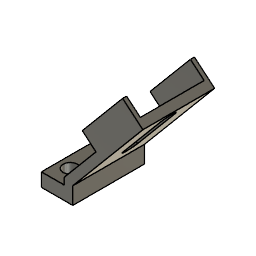
speed_sensor_holder_front_2026 (Autodesk Fusion 360 design; units mm, degrees)
part number: 2026-03-24-16-21-24-312
Autodesk Fusion 360 part; units mm, degrees
sketch "Sketch2" plane through (0, 0, 0) normal (0, 0, 1) x (1, 0, 0)
  line L0 (-7.5122, 7.9259) -> (-0.5122, 7.9259)
  line L1 (-0.5122, 7.9259) -> (-0.5122, -8.0741)
  line L2 (-0.5122, -8.0741) -> (-7.5122, -8.0741)
  line L3 (-7.5122, -8.0741) -> (-7.5122, 7.9259)
  dimension "d1" = 7
  dimension "d2" = 16
  constraint horizontal L0
  constraint vertical L1
  constraint horizontal L2
  constraint vertical L3
  measures "d1" distance of L0.start L0.end
  measures "d2" distance of L0.start L2.end
extrude "Extrude1" add sketch "Sketch2" along normal blind 3 makes body 1
sketch "Sketch4" plane through (0, 0, 3) normal (0, 0, 1) x (-1, 0, 0)
  line L0 (7.5122, 8.0741) -> (0.5122, 8.0741)
  line L1 (0.5122, 8.0741) -> (0.5122, -7.9259)
  line L2 (0.5122, -7.9259) -> (7.5122, -7.9259)
  line L3 (7.5122, -7.9259) -> (7.5122, 8.0741)
  line L4 (0.5122, -7.9259) -> (2.4122, -7.9259)
  line L5 (2.4122, -7.9259) -> (2.4122, 8.0741)
  line L6 (2.4122, 8.0741) -> (0.5122, 8.0741)
  line L7 (0.5122, 8.0741) -> (0.5122, -7.9259)
  dimension "d9" = 1.9
  dimension "d10" = 16
  constraint horizontal L4
  constraint vertical L5
  constraint horizontal L6
  constraint vertical L7
  constraint coincident L1.end L2.start
  measures "d9" distance of L1.end L4.end
  measures "d10" distance of L1.end L0.end
extrude "Extrude3" add sketch "Sketch4" along normal blind 25 separate body contours L0 L1 L2 L4 L5 L6 L7 makes body 2
move_body "Move4" bodies 2 to x (1, 0, 0) y (0, 1, 0) z (0, 0, 1) at (0, 0, 10)
sketch "Sketch11" plane through (0, 0, 3) normal (0, 0, 1) x (-1, 0, 0)
  line L0 (7.5122, 8.0741) -> (0.5122, 8.0741)
  line L1 (0.5122, 8.0741) -> (0.5122, -7.9259)
  line L2 (0.5122, -7.9259) -> (7.5122, -7.9259)
  line L3 (7.5122, -7.9259) -> (7.5122, 8.0741)
  line L4 (0.5122, -7.9259) -> (2.4122, -7.9259)
  line L5 (2.4122, -7.9259) -> (2.4122, 8.0741)
  line L6 (2.4122, 8.0741) -> (0.5122, 8.0741)
  line L7 (0.5122, 8.0741) -> (0.5122, -7.9259)
  dimension "d27" = 1.9
  dimension "d28" = 16
  constraint horizontal L4
  constraint vertical L5
  constraint horizontal L6
  constraint vertical L7
  constraint coincident L1.end L2.start
  measures "d27" distance of L1.end L4.end
  measures "d28" distance of L1.end L0.end
extrude "Extrude6" add sketch "Sketch11" along normal blind 1.5 contours L0 L1 L2 L4 L5 L6 L7 bodies 1
move_face "MoveFace1" by (0, 0, -8.5) 1 faces at (-1.7789, -8.0741, 29.6667) on bodies 2
move_body "Move5" bodies 2 to x (1, 0, 0) y (0, 1, 0) z (0, 0, 1) at (0, 0, -8.5)
move_body "Move6" bodies 2 to x (0.766044, 0, -0.642788) y (0, 1, 0) z (0.642788, 0, 0.766044) at (-3.4569, 0, -0.4977)
combine "Combine2" operation add target body 1 tool bodies 2
sketch "Sketch13" plane through (0, 0, 3) normal (0, 0, 1) x (-1, 0, 0)
  line L0 (2.4122, 8.0741) -> (2.4122, -7.9259)
  line L1 (2.4122, -7.9259) -> (7.5122, -7.9259)
  line L2 (7.5122, -7.9259) -> (7.5122, 8.0741)
  line L3 (7.5122, 8.0741) -> (2.4122, 8.0741)
  circle A0 centre (4.9627, 4.1742) radius 1.45
  dimension "d38" = 2.9
  measures "d38" diameter of A0
extrude "Extrude8" cut sketch "Sketch13" against normal blind 3 contours A0 bodies 1
sketch "Sketch14" plane through (0, 0, 3) normal (0, 0, 1) x (-1, 0, 0)
  circle A0 centre (4.9627, 4.1742) radius 1.45
  line L0 (2.4122, 8.0741) -> (2.4122, -7.9259)
  line L1 (2.4122, -7.9259) -> (7.5122, -7.9259)
  line L2 (7.5122, -7.9259) -> (7.5122, 8.0741)
  line L3 (7.5122, 8.0741) -> (2.4122, 8.0741)
  circle A1 centre (4.962, -4.026) radius 1.6
  dimension "d41" = 3.2
  measures "d41" diameter of A1
extrude "Extrude9" cut sketch "Sketch14" against normal blind 3 contours A1 bodies 1
sketch "Sketch15" plane through (-3.6314, 0, 3.0471) normal (-0.766044, 0, 0.642788) x (0, -1, 0)
  line L0 (-7.9259, 1.8967) -> (8.0741, 1.8967)
  line L1 (8.0741, 1.8967) -> (8.0741, 26.8967)
  line L2 (8.0741, 26.8967) -> (-7.9259, 26.8967)
  line L3 (-7.9259, 26.8967) -> (-7.9259, 1.8967)
  line L4 (8.0741, 26.8967) -> (7.1741, 26.8967)
  line L5 (7.1741, 26.8967) -> (7.1741, 12.8967)
  line L6 (7.1741, 12.8967) -> (8.0741, 12.8967)
  line L7 (8.0741, 12.8967) -> (8.0741, 26.8967)
  dimension "d44" = 0.9
  dimension "d45" = 14
  constraint horizontal L4
  constraint vertical L5
  constraint horizontal L6
  constraint vertical L7
  constraint coincident L1.end L2.start
  measures "d44" distance of L1.end L4.end
  measures "d45" distance of L1.end L6.end
extrude "Extrude10" add sketch "Sketch15" along normal blind 4 contours L1 L2 L4 L5 L6 L7 bodies 1
sketch "Sketch16" plane through (-3.6314, 0, 3.0471) normal (-0.766044, 0, 0.642788) x (0, -1, 0)
  line L0 (7.1741, 12.8967) -> (7.1741, 26.8967)
  line L1 (7.1741, 26.8967) -> (-7.9259, 26.8967)
  line L2 (-7.9259, 26.8967) -> (-7.9259, 1.8967)
  line L3 (-7.9259, 1.8967) -> (8.0741, 1.8967)
  line L4 (8.0741, 1.8967) -> (8.0741, 12.8967)
  line L5 (8.0741, 12.8967) -> (7.1741, 12.8967)
  line L6 (-7.9259, 26.8967) -> (-7.0259, 26.8967)
  line L7 (-7.0259, 26.8967) -> (-7.0259, 12.8967)
  line L8 (-7.0259, 12.8967) -> (-7.9259, 12.8967)
  line L9 (-7.9259, 12.8967) -> (-7.9259, 26.8967)
  dimension "d48" = 0.9
  dimension "d49" = 14
  constraint horizontal L6
  constraint vertical L7
  constraint horizontal L8
  constraint vertical L9
  constraint coincident L1.end L2.start
  measures "d48" distance of L1.end L6.end
  measures "d49" distance of L1.end L8.end
extrude "Extrude11" add sketch "Sketch16" along normal blind 4 contours L1 L2 L6 L7 L8 L9 bodies 1
hole "Hole1" at (-4.9627, -4.1742, 3) direction (0, 0, -1) diameter 3.2 depth 5 tip angle 118 bodies 1
sketch "Sketch17" plane through (-3.6314, 0, 3.0471) normal (-0.766044, 0, 0.642788) x (0, -1, 0)
  line L0 (-7.0259, 26.8967) -> (-7.0259, 12.8967)
  line L1 (-7.0259, 12.8967) -> (-7.9259, 12.8967)
  line L2 (-7.9259, 12.8967) -> (-7.9259, 1.8967)
  line L3 (-7.9259, 1.8967) -> (8.0741, 1.8967)
  line L4 (8.0741, 1.8967) -> (8.0741, 12.8967)
  line L5 (8.0741, 12.8967) -> (7.1741, 12.8967)
  line L6 (7.1741, 12.8967) -> (7.1741, 26.8967)
  line L7 (7.1741, 26.8967) -> (-7.0259, 26.8967)
  line L8 (-1.6, 23) -> (-1.6, 10)
  arc A0 (-1.6, 10) -> (1.6, 10) centre (0, 10) ccw
  line L9 (1.6, 10) -> (1.6, 23)
  arc A1 (1.6, 23) -> (-1.6, 23) centre (0, 23) ccw
  line L10 (0, 23) -> (0, 10) construction
  dimension "d55" = 3.2
  constraint tangent L8 A0
  constraint tangent A0 L9
  constraint parallel L8 L9
  constraint tangent L9 A1
  constraint tangent L8 A1
  constraint parallel L0 L10
  measures "d55" diameter of A0
extrude "Extrude12" cut sketch "Sketch17" against normal blind 4 contours L8 A0 L9 A1 bodies 1
